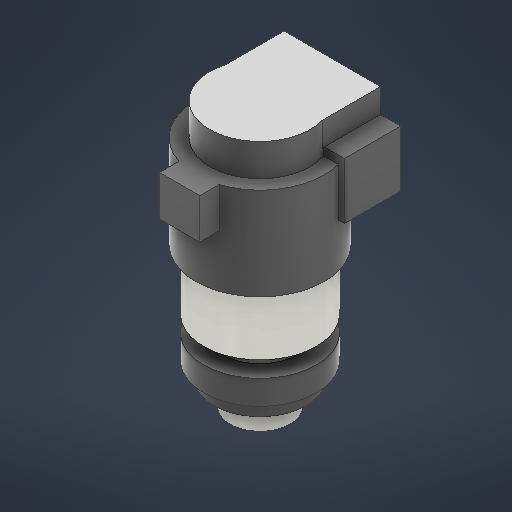
# Autodesk Inventor part: injector carcasa - 3
Saved by Autodesk Inventor 2026.1 (Build 301233000, 233)
## iProperties
Created: 2025-06-10
Part Number: injector carcasa - 3
Material: Generic
Document SubType Name: Sheet Metal
Designer: patri
Density: 1 g/cm^3
Appearance: Default
Sheet Metal Rule: Default
Author: patri
Autodesk Inventor part; units mm, degrees
ref_plane "YZ Plane" through (0, 0, 0) normal (1, 0, 0) x (0, 1, 0)
ref_plane "XZ Plane" through (0, 0, 0) normal (0, 1, 0) x (-1, 0, 0)
ref_plane "XY Plane" through (0, 0, 0) normal (0, 0, 1) x (1, 0, 0)
sketch "Sketch1" plane through (0, 0, 0) normal (0, 1, 0) x (-1, 0, 0)
  circle A0 centre (0, 0) radius 3.75
  dimension "d0" = 7.5
  constraints: 1 centre point, 1 coincident
  measures "d0" diameter of A0
extrude "Extrusion1" add sketch "Sketch1" along normal blind 5
sketch "Sketch2" plane through (0, 5, 0) normal (0, 1, 0) x (1, 0, 0)
  circle A0 centre (0, 0) radius 7
  dimension "d3" = 14
  constraints: 1 centre point, 1 coincident
  measures "d3" diameter of A0
extrude "Extrusion2" add sketch "Sketch2" along normal blind 4
sketch "Sketch3" plane through (0, 9, 0) normal (0, 1, 0) x (1, 0, 0)
  circle A0 centre (0, 0) radius 4.75
  dimension "d6" = 9.5
  constraints: 1 centre point, 1 coincident
  measures "d6" diameter of A0
extrude "Extrusion3" add sketch "Sketch3" along normal blind 4
sketch "Sketch4" plane through (0, 0, 0) normal (1, 0, 0) x (0, 1, 0)
  line L0 (5, -7) -> (5, 7) projected
  line L1 (9, -7) -> (9, 7) projected
  line L2 (13, -4.75) -> (13, 4.75) projected
  line L3 (0, -3.75) -> (0, 3.75) projected
  point P0 (0, 0)
  dimension "d9" = 4
  dimension "d10" = 4
  dimension "d11" = 5
  measures "d9" distance between parallel lines of L0 L1
  measures "d10" distance between parallel lines of L1 L2
  measures "d11" distance between parallel lines of L0 L3
sketch "Sketch5" plane through (0, 13, 0) normal (0, 1, 0) x (1, 0, 0)
  circle A0 centre (0, 0) radius 7
  dimension "d12" = 14
  constraints: 1 centre point, 1 coincident
  measures "d12" diameter of A0
extrude "Extrusion4" add sketch "Sketch5" along normal blind 4.5
sketch "Sketch6" plane through (0, 17.5, 0) normal (0, 1, 0) x (1, 0, 0)
  circle A0 centre (0, 0) radius 8
  dimension "d15" = 16
  constraints: 1 centre point, 1 coincident
  measures "d15" diameter of A0
extrude "Extrusion5" add sketch "Sketch6" along normal blind 11.5
sketch "Sketch7" plane through (0, 29, 0) normal (0, 1, 0) x (1, 0, 0)
  circle A0 centre (0, 0) radius 6.25
  dimension "d18" = 12.5
  constraints: 1 centre point, 1 coincident
  measures "d18" diameter of A0
extrude "Extrusion6" add sketch "Sketch7" along normal blind 25
sketch "Sketch8" plane through (0, 0, 0) normal (1, 0, 0) x (0, 1, 0)
  line L0 (54, -6.25) -> (54, 6.25) projected
  line L1 (0, -3.75) -> (0, 3.75) projected
  line L2 (29, -8) -> (29, 8) projected
  line L3 (17.5, -8) -> (17.5, 8) projected
  point P0 (0, 0)
  point P1 (0, 0)
  dimension "d21" = 54
  dimension "d22" = 29
  dimension "d23" = 17.5
  constraints: 1 midpoint
  measures "d21" distance between parallel lines of L0 L1
  measures "d22" distance from line of L2 point (0, 0)
  measures "d23" distance from line of L3 point (0, 0)
sketch "Sketch9" plane through (0, 54, 0) normal (0, 1, 0) x (1, 0, 0)
  circle A0 centre (0, 0) radius 7
  dimension "d24" = 14
  constraints: 1 centre point, 1 coincident
  measures "d24" diameter of A0
extrude "Extrusion7" add sketch "Sketch9" along normal blind 10
sketch "Sketch10" plane through (0, 0, 0) normal (1, 0, 0) x (0, 1, 0)
  line L0 (64, -7) -> (64, 7) projected
  line L1 (0, -3.75) -> (0, 3.75) projected
  point P0 (0, 0)
  dimension "d27" = 64
  measures "d27" distance between parallel lines of L0 L1
sketch "Sketch11" plane through (0, 64, 0) normal (0, 1, 0) x (1, 0, 0)
  circle A0 centre (0, 0) radius 7
  dimension "d28" = 14
  constraints: 1 centre point, 1 coincident
  measures "d28" diameter of A0
extrude "Extrusion8" add sketch "Sketch11" along normal blind 9
sketch "Sketch12" plane through (0, 73, 0) normal (0, 1, 0) x (1, 0, 0)
  circle A0 centre (0, 0) radius 4.5
  dimension "d31" = 9
  constraints: 1 centre point, 1 coincident
  measures "d31" diameter of A0
extrude "Extrusion9" add sketch "Sketch12" along normal blind 1
sketch "Sketch13" plane through (0, 0, 0) normal (1, 0, 0) x (0, 1, 0)
  point P0 (0, 0)
sketch "Sketch14" plane through (0, 0, 0) normal (1, 0, 0) x (0, 1, 0)
  line L0 (73, -7) -> (73, 7) projected
  line L1 (0, -3.75) -> (0, 3.75) projected
  line L2 (74, -4.5) -> (74, 4.5) projected
  point P0 (0, 0)
  point P1 (0, 0)
  dimension "d34" = 73
  dimension "d35" = 74
  constraints: 1 midpoint
  measures "d34" distance between parallel lines of L0 L1
  measures "d35" distance from line of L2 point (0, 0)
sketch "Sketch15" plane through (0, 74, 0) normal (0, 1, 0) x (1, 0, 0)
  circle A0 centre (0, 0) radius 7
  dimension "d36" = 14
  constraints: 1 centre point, 1 coincident
  measures "d36" diameter of A0
extrude "Extrusion10" add sketch "Sketch15" along normal blind 11.5
sketch "Sketch16" plane through (0, 0, 0) normal (1, 0, 0) x (0, 1, 0)
  line L0 (85.5, -7) -> (85.5, 7) projected
  line L1 (0, -3.75) -> (0, 3.75) projected
  point P0 (0, 0)
  dimension "d39" = 85.5
  measures "d39" distance between parallel lines of L0 L1
sketch "Sketch17" plane through (0, 0, 0) normal (1, 0, 0) x (0, 1, 0)
  line L0 (23, -9) -> (30, -9)
  line L1 (0, -3.75) -> (0, 3.75) projected
  line L2 (23, -9) -> (23, -2)
  line L3 (54, 7) -> (73, 7) projected
  line L4 (23, -2) -> (30, -2)
  line L5 (30, -2) -> (30, -9)
  point P0 (0, 0)
  point P1 (0, 0)
  point P2 (26.5, -9)
  dimension "d40" = 7
  dimension "d41" = 23
  dimension "d42" = 7
  dimension "d43" = 9
  constraints: 8 end point, 3 perpendicular, 2 midpoint, 1 horizontal
  measures "d40" distance of L0.start L0.end
  measures "d41" distance from line of L0.start L1
  measures "d42" distance of L0.start L2.end
  measures "d43" vertical distance of point (0, 0) point (26.5, -9)
extrude "Extrusion11" add sketch "Sketch17" along normal mid plane 17
sketch "Sketch18" plane through (0, 0, 0) normal (1, 0, 0) x (0, 1, 0)
  line L0 (24, 10) -> (29, 10)
  line L1 (29, 10) -> (29, 6)
  line L2 (29, 6) -> (24, 6)
  line L3 (17.5, 8) -> (29, 8) projected
  line L4 (24, 6) -> (24, 10)
  line L5 (0, -3.75) -> (0, 3.75) projected
  point P0 (0, 0)
  point P1 (24, 8)
  point P2 (0, 0)
  point P3 (26.5, 10)
  dimension "d46" = 5
  dimension "d47" = 4
  dimension "d48" = 24
  dimension "d49" = 10
  constraints: 8 end point, 3 midpoint, 2 perpendicular, 1 horizontal, 1 parallel
  measures "d46" distance of L0.start L0.end
  measures "d47" distance of L0.end L1.end
  measures "d48" distance from line of L5 point (24, 8)
  measures "d49" vertical distance of point (0, 0) point (26.5, 10)
extrude "Extrusion12" add sketch "Sketch18" along normal mid plane 5
sketch "Sketch19" plane through (8.5, 0, 0) normal (1, 0, 0) x (0, 0, -1)
  line L0 (3.75, 0) -> (-3.75, 0) projected
  point P0 (0, 0)
  point P1 (9, 23)
  dimension "d52" = 23
  measures "d52" distance from line of point (9, 23) L0
sketch "Sketch20" plane through (8.5, 30, -9) normal (0, 0, -1) x (-1, 0, 0)
  line L0 (14.4214, 0) -> (2.5786, 0) projected
  line L1 (8.5, 0) -> (2.5, 0)
  line L2 (2.5, 0) -> (2.5, 29)
  line L3 (1.5, 24) -> (1.5, 43) projected
  line L4 (2.5, 29) -> (14.5, 29)
  line L5 (14.5, 29) -> (14.5, 0)
  line L6 (14.5, 0) -> (2.5, 0)
  point P0 (8.5, -30)
  point P1 (2.5786, 0)
  dimension "d53" = 6
  dimension "d54" = 29
  dimension "d55" = 90
  dimension "d56" = 12
  dimension "d57" = 29
  dimension "d58" = 90
  constraints: 10 end point, 2 perpendicular, 1 collinear, 1 midpoint, 1 parallel
  measures "d53" distance of L1.start L1.end
  measures "d54" distance of L1.end L2.end
  measures "d55" angle of L1 L2
  measures "d56" distance of L2.end L4.end
  measures "d57" distance of L4.end L5.end
  measures "d58" angle of L4 L5
extrude "Extrusion13" add sketch "Sketch20" against normal blind 9
sketch "Sketch21" plane through (8.5, 23, -9) normal (0, 0, -1) x (-1, 0, 0)
  point P0 (8.5, -23)
sketch "Sketch22" plane through (0, 13, 0) normal (0, -1, 0) x (1, 0, 0)
  circle A0 centre (0, 0) radius 7
  constraints: 1 centre point, 1 coincident
extrude "Extrusion14" add sketch "Sketch22" along normal blind 3
sketch "Sketch23" plane through (0, 9, 0) normal (0, 1, 0) x (1, 0, 0)
  circle A0 centre (0, 0) radius 3.75 projected
  circle A1 centre (0, 0) radius 7
  circle A2 centre (0, 0) radius 7
  circle A3 centre (0, 0) radius 4.75
  dimension "d63" = 14
  dimension "d64" = 9.5
  constraints: 3 centre point, 3 coincident, 1 concentric
  measures "d63" diameter of A1
  measures "d64" diameter of A3
extrude "Extrusion15" cut sketch "Sketch23" against normal blind 1 contours A1
sketch "Sketch24" plane through (0, 5, 0) normal (0, -1, 0) x (1, 0, 0)
  circle A0 centre (0, 0) radius 5.75
  dimension "d67" = 11.5
  constraints: 1 centre point, 1 coincident
  measures "d67" diameter of A0
extrude "Extrusion16" add sketch "Sketch24" along normal blind 2
sketch "Sketch25" plane through (0, 85.5, 0) normal (0, 1, 0) x (1, 0, 0)
  circle A0 centre (0, 0) radius 7
  constraints: 1 centre point, 1 coincident
extrude "Extrusion17" cut sketch "Sketch25" against normal blind 6.5
sketch "Sketch26" plane through (0, 0, 0) normal (1, 0, 0) x (0, 1, 0)
  line L0 (79, 7) -> (79, -7) projected
  line L1 (0, -3.75) -> (0, 3.75) projected
  point P0 (0, 0)
  dimension "d72" = 79
  measures "d72" distance between parallel lines of L0 L1
sketch "Sketch27" plane through (0, 79, 0) normal (0, 1, 0) x (1, 0, 0)
  point P0 (0, 0)
sketch "Sketch28" plane through (0, 79, 0) normal (0, 1, 0) x (1, 0, 0)
  circle A0 centre (0, 0) radius 17.2984
  constraints: 1 centre point, 1 coincident
extrude "Extrusion18" cut sketch "Sketch28" against normal blind 13
extrude "Extrusion19" cut sketch "Sketch28" against normal blind 46
equation "\"BendRadius\" = Thickness"
equation "\"BendReliefWidth\" = Thickness"
equation "\"BendReliefDepth\" = 0.5 * Thickness"
equation "\"CornerReliefSize\" = 4 * Thickness"
equation "\"MinimumRemnant\" = 2 * Thickness"
equation "\"TransitionRadius\" = BendRadius"
equation "\"JacobiRadiusSize\" = BendRadius"
equation "\"GapSize\" = Thickness"
equation "\"Thickness\" = 3.048"
body "Solid1"
